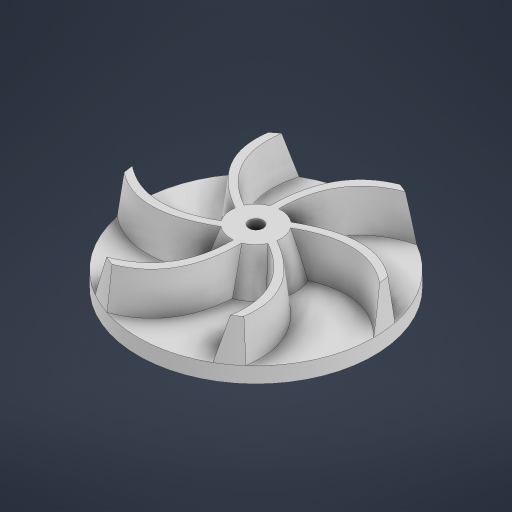
# Autodesk Inventor part: Fan
Saved by Autodesk Inventor 2023 (Build 270158000, 158)
## iProperties
Created: 2022-03-30
Part Number: Fan
Material: 一般
Document SubType Name: Modeling
Designer: neko2
Density: 1 g/cm^3
Appearance: 既定
Author: neko2
Autodesk Inventor part; units mm, degrees
ref_plane "YZ Plane" through (0, 0, 0) normal (1, 0, 0) x (0, 1, 0)
ref_plane "XZ Plane" through (0, 0, 0) normal (0, 1, 0) x (-1, 0, 0)
ref_plane "XY Plane" through (0, 0, 0) normal (0, 0, 1) x (1, 0, 0)
sketch "スケッチ1" plane through (0, 0, 0) normal (0, 1, 0) x (-1, 0, 0)
  circle A0 centre (0, 0) radius 7.5
  dimension "d0" = 15
  constraints: 1 centre point, 1 coincident
  measures "d0" diameter of A0
extrude "押し出し1" add sketch "スケッチ1" along normal blind 1
sketch "スケッチ3" plane through (0, 1, 0) normal (0, 1, 0) x (1, 0, 0)
  line L0 (0.5, 0) -> (4.5, 3) construction
  line L1 (4.5, 3) -> (7.5, 0) construction
  spline S0 degree 2 poles (0.5, 0) (4.5, 3) (7.5, 0) knots 1 1 1 2 2 2
  line L2 (0.5, 1.3) -> (4.5, 3.8) construction
  line L3 (4.5, 3.8) -> (7.348469, 1.5) construction
  spline S1 degree 2 poles (0.5, 1.3) (4.5, 3.8) (7.348469, 1.5) knots 1 1 1 2 2 2
  line L4 (0.5, 0) -> (0.5, 1.3)
  line L5 (4.5, 3) -> (4.5, 3.8)
  circle A0 centre (0, 0) radius 7.5
  line L6 (0.25, 0.433013) -> (-0.348076, 5.397114) construction
  line L7 (-0.348076, 5.397114) -> (3.75, 6.495191) construction
  spline S2 degree 2 poles (0.25, 0.433013) (-0.348076, 5.397114) (3.75, 6.495191) knots 1 1 1 2 2 2
  spline S3 degree 2 poles (-0.875833, 1.083013) (-1.040897, 5.797114) (2.375197, 7.113961) knots 1 1 1 2 2 2
  line L8 (-0.875833, 1.083013) -> (-1.040897, 5.797114) construction
  line L9 (-1.040897, 5.797114) -> (2.375197, 7.113961) construction
  line L10 (0.25, 0.433013) -> (-0.875833, 1.083013)
  line L11 (-0.348076, 5.397114) -> (-1.040897, 5.797114)
  line L12 (-0.25, 0.433013) -> (-4.848076, 2.397114) construction
  line L13 (-4.848076, 2.397114) -> (-3.75, 6.495191) construction
  spline S4 degree 2 poles (-0.25, 0.433013) (-4.848076, 2.397114) (-3.75, 6.495191) knots 1 1 1 2 2 2
  spline S5 degree 2 poles (-1.375833, -0.216987) (-5.540897, 1.997114) (-4.973273, 5.613961) knots 1 1 1 2 2 2
  line L14 (-1.375833, -0.216987) -> (-5.540897, 1.997114) construction
  line L15 (-5.540897, 1.997114) -> (-4.973273, 5.613961) construction
  line L16 (-0.25, 0.433013) -> (-1.375833, -0.216987)
  line L17 (-4.848076, 2.397114) -> (-5.540897, 1.997114)
  line L18 (-0.5, 0) -> (-4.5, -3) construction
  line L19 (-4.5, -3) -> (-7.5, 0) construction
  spline S6 degree 2 poles (-0.5, 0) (-4.5, -3) (-7.5, 0) knots 1 1 1 2 2 2
  spline S7 degree 2 poles (-0.5, -1.3) (-4.5, -3.8) (-7.348469, -1.5) knots 1 1 1 2 2 2
  line L20 (-0.5, -1.3) -> (-4.5, -3.8) construction
  line L21 (-4.5, -3.8) -> (-7.348469, -1.5) construction
  line L22 (-0.5, 0) -> (-0.5, -1.3)
  line L23 (-4.5, -3) -> (-4.5, -3.8)
  line L24 (-0.25, -0.433013) -> (0.348076, -5.397114) construction
  line L25 (0.348076, -5.397114) -> (-3.75, -6.495191) construction
  spline S8 degree 2 poles (-0.25, -0.433013) (0.348076, -5.397114) (-3.75, -6.495191) knots 1 1 1 2 2 2
  spline S9 degree 2 poles (0.875833, -1.083013) (1.040897, -5.797114) (-2.375197, -7.113961) knots 1 1 1 2 2 2
  line L26 (0.875833, -1.083013) -> (1.040897, -5.797114) construction
  line L27 (1.040897, -5.797114) -> (-2.375197, -7.113961) construction
  line L28 (-0.25, -0.433013) -> (0.875833, -1.083013)
  line L29 (0.348076, -5.397114) -> (1.040897, -5.797114)
  line L30 (0.25, -0.433013) -> (4.848076, -2.397114) construction
  line L31 (4.848076, -2.397114) -> (3.75, -6.495191) construction
  spline S10 degree 2 poles (0.25, -0.433013) (4.848076, -2.397114) (3.75, -6.495191) knots 1 1 1 2 2 2
  spline S11 degree 2 poles (1.375833, 0.216987) (5.540897, -1.997114) (4.973273, -5.613961) knots 1 1 1 2 2 2
  line L32 (1.375833, 0.216987) -> (5.540897, -1.997114) construction
  line L33 (5.540897, -1.997114) -> (4.973273, -5.613961) construction
  line L34 (0.25, -0.433013) -> (1.375833, 0.216987)
  line L35 (4.848076, -2.397114) -> (5.540897, -1.997114)
  point P0 (3.75, 6.495191)
  point P1 (2.375197, 7.113961)
  point P2 (-3.75, 6.495191)
  point P3 (-4.973273, 5.613961)
  point P4 (-7.5, 0)
  point P5 (-7.348469, -1.5)
  point P6 (-3.75, -6.495191)
  point P7 (-2.375197, -7.113961)
  point P8 (3.75, -6.495191)
  point P9 (4.973273, -5.613961)
  dimension "d4" = 3
  dimension "d5" = 2.5
  dimension "d6" = 1.3
  dimension "d8" = 0.5
  dimension "d10" = 1.5
  dimension "d11" = 3
  dimension "d14" = 360
  constraints: 24 end point, 12 coincident, 2 horizontal alignment, 2 point on circle, 2 vertical, 133 other
  measures "d4" vertical distance of L0.end L0.start
  measures "d5" vertical distance of L2.end L2.start
  measures "d6" distance of L0.start L2.start
  measures "d8" distance from line of L4 point (0, 0)
  measures "d10" vertical distance of L3.end L1.end
  measures "d11" horizontal distance of L1.end L0.end
sketch "スケッチ3 outline for 押し出し2" plane through (0, 1, 0) normal (0, 1, 0) x (1, 0, 0)
  line L0 (0.5, 1.3) -> (0.5, 0)
  spline S0 degree 2 poles (0.5, 1.3) (4.5, 3.8) (7.348469, 1.5) knots 0 0 0 1 1 1
  arc A0 (7.5, 0) -> (7.348469, 1.5) centre (0, 0) ccw
  spline S1 degree 2 poles (0.5, 0) (4.5, 3) (7.5, 0) knots 0 0 0 1 1 1
  line L1 (1.375833, 0.216987) -> (0.25, -0.433013)
  spline S2 degree 2 poles (1.375833, 0.216987) (5.540897, -1.997114) (4.973273, -5.613961) knots 0 0 0 1 1 1
  arc A1 (3.75, -6.495191) -> (4.973273, -5.613961) centre (0, 0) ccw
  spline S3 degree 2 poles (0.25, -0.433013) (4.848076, -2.397114) (3.75, -6.495191) knots 0 0 0 1 1 1
  line L2 (-0.875833, 1.083013) -> (0.25, 0.433013)
  spline S4 degree 2 poles (-0.875833, 1.083013) (-1.040897, 5.797114) (2.375197, 7.113961) knots 0 0 0 1 1 1
  arc A2 (3.75, 6.495191) -> (2.375197, 7.113961) centre (0, 0) ccw
  spline S5 degree 2 poles (0.25, 0.433013) (-0.348076, 5.397114) (3.75, 6.495191) knots 0 0 0 1 1 1
  line L3 (-1.375833, -0.216987) -> (-0.25, 0.433013)
  spline S6 degree 2 poles (-1.375833, -0.216987) (-5.540897, 1.997114) (-4.973273, 5.613961) knots 0 0 0 1 1 1
  arc A3 (-3.75, 6.495191) -> (-4.973273, 5.613961) centre (0, 0) ccw
  spline S7 degree 2 poles (-0.25, 0.433013) (-4.848076, 2.397114) (-3.75, 6.495191) knots 0 0 0 1 1 1
  line L4 (-0.5, -1.3) -> (-0.5, 0)
  spline S8 degree 2 poles (-0.5, -1.3) (-4.5, -3.8) (-7.348469, -1.5) knots 0 0 0 1 1 1
  arc A4 (-7.5, 0) -> (-7.348469, -1.5) centre (0, 0) ccw
  spline S9 degree 2 poles (-0.5, 0) (-4.5, -3) (-7.5, 0) knots 0 0 0 1 1 1
  line L5 (0.875833, -1.083013) -> (-0.25, -0.433013)
  spline S10 degree 2 poles (0.875833, -1.083013) (1.040897, -5.797114) (-2.375197, -7.113961) knots 0 0 0 1 1 1
  arc A5 (-3.75, -6.495191) -> (-2.375197, -7.113961) centre (0, 0) ccw
  spline S11 degree 2 poles (-0.25, -0.433013) (0.348076, -5.397114) (-3.75, -6.495191) knots 0 0 0 1 1 1
extrude "押し出し2" add sketch "スケッチ3 outline for 押し出し2" along normal blind 2.5 draft -7
sketch "スケッチ4" plane through (0, 1, 0) normal (0, 1, 0) x (1, 0, 0)
  circle A0 centre (0, 0) radius 2.5
  dimension "d18" = 5
  constraints: 1 centre point, 1 coincident
  measures "d18" diameter of A0
extrude "押し出し3" add sketch "スケッチ4" along normal blind 2.5 draft -20
sketch "スケッチ5" plane through (0, 3.5, 0) normal (0, 1, 0) x (1, 0, 0)
  arc A0 (-0.850704, 2.350809) -> (-2.046217, 1.436313) centre (0, 0) ccw
  circle A1 centre (0, 0) radius 0.45
  dimension "d21" = 0.9
  constraints: 1 centre point, 1 coincident
  measures "d21" diameter of A1
extrude "押し出し4" cut sketch "スケッチ5" against normal through all
